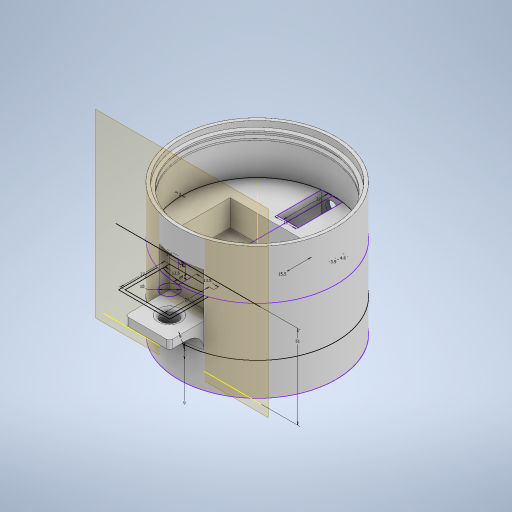
# Autodesk Inventor part: final_탄두_middle
Saved by Autodesk Inventor 2023 (Build 270158000, 158)
## iProperties
Created: 2023-10-31
Part Number: final_탄두_middle
Material: 일반
Document SubType Name: Modeling
Designer: rlatk
Density: 1 g/cm^3
Appearance: 기본값
Author: rlatk
Autodesk Inventor part; units mm, degrees
ref_plane "YZ Plane" through (0, 0, 0) normal (1, 0, 0) x (0, 1, 0)
ref_plane "XZ Plane" through (0, 0, 0) normal (0, 1, 0) x (-1, 0, 0)
sketch "스케치1" plane through (0, 0, 0) normal (0, 1, 0) x (-1, 0, 0)
  circle A0 centre (0, 0) radius 45.85
  circle A1 centre (0, 0) radius 47.85
  dimension "d0" = 91.7
  dimension "d1" = 2
  constraints: 2 centre point, 1 coincident
  measures "d0" diameter of A0
  measures "d1" radial gap between concentric circles of A0 A1
extrude "돌출1" add sketch "스케치1" along normal blind 10
ref_plane "작업 평면1" through (0, 0, 45.75) normal (0, 0, 1) x (1, 0, 0)
sketch "스케치2" plane through (0, 0, 45.75) normal (0, 0, 1) x (1, 0, 0)
  circle A0 centre (0, 9) radius 4.5
  line L0 (47.85, 0) -> (-47.85, 0) projected
  line L1 (-40.336, 51) -> (47.75, 51)
  line L2 (2, 52.9) -> (-2, 52.9)
  line L3 (-2, 52.9) -> (-2, 49.1)
  line L4 (-2, 49.1) -> (2, 49.1)
  line L5 (2, 49.1) -> (2, 52.9)
  line L6 (2, 52.9) -> (-2, 49.1) construction
  line L7 (-2, 52.9) -> (2, 49.1) construction
  point P0 (0, 0)
  point P1 (0, 51)
  dimension "d5" = 9
  dimension "d6" = 9
  dimension "d10" = 51
  dimension "d11" = 4
  dimension "d12" = 3.8
  constraints: 14 end point, 2 horizontal, 2 midpoint, 2 parallel, 1 centre point, 1 perpendicular, 1 point on line
  measures "d5" diameter of A0
  measures "d6" distance from line of L0 A0.centre
  measures "d10" distance between parallel lines of L1 L0
  measures "d11" distance of L4.end L3.end
  measures "d12" distance of L3.end L2.end
sketch "스케치3" plane through (0, 0, 0) normal (1, 0, 0) x (0, 1, 0)
  line L0 (10, 45.85) -> (0, 45.85) projected
  line L1 (-22.58, 0) -> (65.48, 0) projected
  line L2 (10, 45.85) -> (0, 45.85) projected
  line L3 (52.9, 45.85) -> (49.1, 45.85)
  line L4 (49.1, 45.85) -> (49.1, 44.85)
  line L5 (49.1, 44.85) -> (52.9, 44.85)
  line L6 (52.9, 44.85) -> (52.9, 45.85)
  point P0 (0, 0)
  point P1 (49.1, 45.75)
  point P2 (49.1, 45.75)
  point P3 (49.1, 45.75)
  point P4 (52.9, 45.75)
  point P5 (52.9, 45.75)
  point P6 (52.9, 45.75)
  dimension "d17" = 1
  constraints: 8 end point, 2 parallel, 1 horizontal, 1 perpendicular, 1 point on line, 1 other
  measures "d17" distance of L4.end L3.end
sketch "스케치4" plane through (0, 0, 0) normal (0, -1, 0) x (1, 0, 0)
  point P0 (0, 0)
sketch "스케치5" plane through (0, 0, 0) normal (0, -1, 0) x (1, 0, 0)
  circle A0 centre (0, 0) radius 45.85 projected
  circle A1 centre (0, 0) radius 47.85 projected
  circle A2 centre (0, 0) radius 45.85
  circle A3 centre (0, 0) radius 47.85
  constraints: 2 centre point, 2 coincident, 2 concentric
extrude "돌출4" add sketch "스케치5" along normal blind 10
sketch "스케치6" plane through (0, 0, 45.75) normal (0, 0, 1) x (1, 0, 0)
  point P0 (0, 0)
sketch "스케치7" plane through (0, 0, 0) normal (1, 0, 0) x (0, 1, 0)
  line L0 (10, 45.85) -> (-10, 45.85) projected
  line L1 (-9, 45.85) -> (-7, 45.85)
  line L2 (-7, 45.85) -> (-7, 43.85)
  line L3 (-7, 43.85) -> (-9, 43.85)
  line L4 (-9, 43.85) -> (-9, 45.85)
  line L5 (-9, 45.85) -> (-8.5, 43.85)
  line L6 (-7, 45.85) -> (-7.5, 43.85)
  point P0 (0, 0)
  dimension "d21" = 2
  dimension "d22" = 2
  dimension "d23" = 1
  dimension "d24" = 0.5
  dimension "d25" = 0.5
  constraints: 12 end point, 3 point on line, 2 parallel, 1 horizontal, 1 perpendicular
  measures "d21" distance of L2.end L3.end
  measures "d22" distance of L1.end L2.end
  measures "d23" distance of L1.start L0.end
  measures "d24" distance of L5.end L3.end
  measures "d25" distance of L2.end L6.end
coil "코일1" sketch "스케치7" operation add axis through (0, -10, 0) along (0, 1, 0) pitch 4 turns 2 hand right contours L6 L3 L5 L0
sketch "스케치8" plane through (0, 0, 0) normal (0, 0, 1) x (1, 0, 0)
  line L0 (-47.85, -10) -> (47.85, -10) projected
  line L1 (47.85, 10) -> (-47.85, 10) projected
  point P0 (0, 0)
sketch "스케치9" plane through (0, 10, 0) normal (0, 1, 0) x (1, 0, 0)
  circle A0 centre (0, 0) radius 47.85 projected
  circle A1 centre (0, 0) radius 45.85 projected
  circle A2 centre (0, 0) radius 47.85
  constraints: 1 centre point, 1 coincident, 1 concentric
extrude "돌출5" add sketch "스케치9" along normal blind 30 contours A0 | A1
sketch "스케치10" plane through (0, 40, 0) normal (0, 1, 0) x (1, 0, 0)
  circle A0 centre (0, 0) radius 47.85 projected
  circle A1 centre (0, 0) radius 45.85
  circle A2 centre (0, 0) radius 47.85
  line L0 (0, -47.85) -> (0, 47.85)
  line L1 (-6.5, 45.3869) -> (-6.5, 18.3869)
  line L2 (-6.5, 18.3869) -> (6.5, 18.3869)
  circle A3 centre (0, 0) radius 45.85 projected
  line L3 (0, 45.85) -> (-0.1096, 45.3869) construction
  line L4 (0, 45.85) -> (0.1096, 45.3869) construction
  line L5 (-6.5, 45.3869) -> (6.5, 45.3869)
  line L6 (6.5, 18.3869) -> (6.5, 45.3869)
  dimension "d36" = 2
  dimension "d37" = 13
  dimension "d39" = 27
  constraints: 14 end point, 5 point on circle, 3 point on line, 2 centre point, 1 coincident, 1 parallel, 1 vertical
  measures "d36" radial gap between concentric circles of A0 A1
  measures "d37" distance of L2.end L1.end
  measures "d39" distance between parallel lines of L5 L2
extrude "돌출6" cut sketch "스케치10" against normal blind 27 contours L6 L2 L0 L5 | L5 L0 L2 L1
sketch "스케치11" plane through (0, 13, 0) normal (0, 1, 0) x (1, 0, 0)
  line L0 (-6.5, 45.3869) -> (6.5, 45.3869) projected
  line L1 (-6.5, 18.3869) -> (-6.5, 45.3869) projected
  line L2 (6.5, 18.3869) -> (-6.5, 18.3869) projected
  line L3 (6.5, 45.3869) -> (6.5, 18.3869) projected
  line L4 (-6.5, 18.3869) -> (-6.5, 45.3869) projected
  line L5 (-6.5, 45.3869) -> (6.5, 45.3869)
  line L6 (6.5, 45.3869) -> (6.5, 40.7869)
  line L7 (6.5, 40.7869) -> (-6.5, 40.7869)
  line L8 (-6.5, 40.7869) -> (-6.5, 45.3869)
  line L9 (-6.5, 33.8869) -> (6.5, 33.8869)
  line L10 (-6.5, 36.8869) -> (6.5, 36.8869)
  point P0 (0, 0)
  dimension "d42" = 4.6
  dimension "d43" = 15.5
  dimension "d44" = 3.9
  constraints: 12 end point, 5 point on line, 3 perpendicular, 2 parallel, 1 horizontal
  measures "d42" distance of L5.end L6.end
  measures "d43" distance between parallel lines of L2 L9
  measures "d44" distance between parallel lines of L10 L7
extrude "돌출10" add sketch "스케치9" against normal blind 5 contours A1
extrude "돌출12" cut sketch "스케치11" against normal blind 5.2 contours L10 L3 L9 L1
extrude "돌출13" add sketch "스케치11" along normal blind 7.8 contours L0 L3 L7 L1
sketch "스케치12" plane through (-6.5, 40, -45.3869) normal (0, 0, 1) x (1, 0, 0)
  point P0 (6.5, -40)
sketch "스케치13" plane through (-6.5, 40, -45.3869) normal (0, 0, 1) x (1, 0, 0)
  line L0 (54.35, 0) -> (-41.35, 0) projected
  line L1 (-41.35, -50) -> (54.35, -50) projected
  line L2 (0, -19.2) -> (13, -19.2) projected
  line L3 (13, 0) -> (13, -19.2) projected
  line L4 (0, 0) -> (13, 0) projected
  line L5 (0, 0) -> (0, -19.2) projected
  line L6 (0, -19.2) -> (13, -19.2) projected
  line L7 (0, -19.2) -> (13, -19.2) projected
  line L8 (13, -27) -> (0, -27) projected
  line L9 (13, -19.2) -> (13, -27) projected
  line L10 (0, -19.2) -> (13, -19.2) projected
  line L11 (0, -27) -> (0, -19.2) projected
  circle A0 centre (6.5, -6.3) radius 3.7
  point P0 (6.5, -40)
  dimension "d59" = 7.4
  dimension "d60" = 6.3
  constraints: 1 centre point
  measures "d59" diameter of A0
  measures "d60" distance from line of A0.centre L0
extrude "돌출14" cut sketch "스케치13" against normal blind 7.8 contours A0
sketch "스케치14" plane through (0, 40, 0) normal (0, 1, 0) x (1, 0, 0)
  line L0 (-6.5, 18.3869) -> (-6.5, 45.3869) projected
  line L1 (-6.5, 45.3869) -> (6.5, 45.3869) projected
  line L2 (6.5, 45.3869) -> (6.5, 18.3869) projected
  line L3 (6.5, 18.3869) -> (-6.5, 18.3869) projected
  circle A0 centre (0, 0) radius 47.85 projected
  line L4 (0, 0) -> (0, -47.85)
  line L5 (30, 13.5566) -> (-30, 13.5566)
  line L6 (-30, 13.5566) -> (-30, -26.4434)
  line L7 (-30, -26.4434) -> (30, -26.4434)
  line L8 (30, -26.4434) -> (30, 13.5566)
  line L9 (30, 13.5566) -> (-30, -26.4434) construction
  line L10 (-30, 13.5566) -> (30, -26.4434) construction
  point P0 (0, -6.4434)
  dimension "d63" = 60
  dimension "d64" = 40
  constraints: 14 end point, 2 midpoint, 2 parallel, 1 horizontal, 1 perpendicular, 1 point on line, 1 vertical alignment, 1 other
  measures "d63" distance of L7.end L6.end
  measures "d64" distance of L6.end L5.end
extrude "돌출15" cut sketch "스케치14" against normal blind 16 contours L8 L7 L6 L5
extrude "돌출16" add sketch "스케치10" along normal blind 30 contours A0 L0 A1 | L0 A1 A0
sketch "스케치15" plane through (0, 0, 45.75) normal (0, 0, 1) x (1, 0, 0)
  point P0 (0, 0)
sketch "스케치16" plane through (0, 0, 0) normal (1, 0, 0) x (0, 1, 0)
  line L0 (5, -45.85) -> (5, 45.85) projected
  line L1 (-1, 45.85) -> (1, 45.85) projected
  line L2 (-7, 45.85) -> (-9, 45.85) projected
  line L3 (-10, -45.85) -> (-10, 45.85) projected
  line L4 (70, 45.85) -> (40, 45.85) projected
  line L5 (58, 45.85) -> (58, 43.85)
  line L6 (58, 43.85) -> (60, 43.85)
  line L7 (60, 43.85) -> (60, 45.85)
  line L8 (59, 45.85) -> (58, 43.85) construction
  line L9 (59, 45.85) -> (60, 43.85) construction
  line L10 (60, 45.85) -> (58, 45.85)
  line L11 (60, 45.85) -> (59.5, 43.85)
  line L12 (58, 45.85) -> (58.5, 43.85)
  point P0 (0, 0)
  dimension "d69" = 11
  dimension "d70" = 2
  dimension "d72" = 0.5
  dimension "d73" = 0.5
  constraints: 16 end point, 3 point on line, 2 horizontal alignment, 1 midpoint, 1 parallel
  measures "d69" distance of L8.start L4.start
  measures "d70" distance of L6.end L5.end
  measures "d72" distance of L5.end L12.end
  measures "d73" distance of L11.end L6.end
coil "코일2" sketch "스케치16" operation add axis through (0, -10, 0) along (0, 1, 0) pitch 4 turns 2 hand right contours L11 L6 L12 L4
sketch "스케치17" plane through (0, 70, 0) normal (0, 1, 0) x (1, 0, 0)
  point P0 (0, 0)
sketch "스케치18" plane through (0, -10, 0) normal (0, -1, 0) x (1, 0, 0)
  circle A0 centre (0, 0) radius 47.85 projected
  circle A1 centre (0, 0) radius 45.85 projected
  circle A2 centre (0, 0) radius 47.85
  circle A3 centre (0, 0) radius 45.85
  constraints: 2 centre point, 2 coincident, 1 concentric
sketch "스케치19" plane through (0, 40, 0) normal (0, 1, 0) x (1, 0, 0)
  circle A0 centre (0, 0) radius 45.85 projected
  circle A1 centre (0, 0) radius 47.85 projected
  line L0 (0, -47.85) -> (0, 47.85) projected
  line L1 (0, -47.85) -> (0, -39.85)
  line L2 (0, -39.85) -> (-13.5, -39.85)
  line L3 (0, -39.85) -> (13.5, -39.85)
  line L4 (-13.5, -39.85) -> (-13.5, -66.85)
  line L5 (13.5, -39.85) -> (13.5, -66.85)
  line L6 (13.5, -66.85) -> (-13.5, -66.85)
  line L7 (-15.5, -68.85) -> (-15.5, -37.85)
  line L8 (-15.5, -37.85) -> (0, -37.85)
  line L9 (0, -37.85) -> (15.5, -37.85)
  line L10 (15.5, -37.85) -> (15.5, -68.85)
  line L11 (15.5, -68.85) -> (-15.5, -68.85)
  circle A2 centre (0, -53.35) radius 5
  point P0 (13.5, -45.9061)
  point P1 (-13.5, -45.9061)
  point P2 (-13.5, -43.8175)
  point P3 (13.5, -43.8175)
  point P4 (-15.5, -43.1506)
  point P5 (15.5, -43.1506)
  dimension "d82" = 8
  dimension "d83" = 13.5
  dimension "d84" = 13.5
  dimension "d85" = 27
  dimension "d86" = 27
  dimension "d87" = 2
  dimension "d88" = 10
  constraints: 22 end point, 2 vertical, 1 centre point, 1 horizontal, 1 perpendicular, 1 point on line, 4 other
  measures "d82" distance of L0.start L1.end
  measures "d83" distance of L1.end L2.end
  measures "d84" distance of L1.end L3.end
  measures "d85" distance of L2.end L4.end
  measures "d86" distance of L3.end L5.end
  measures "d87" distance between parallel lines of L4 L7
  measures "d88" diameter of A2
extrude "돌출18" cut sketch "스케치19" along normal blind 13.5 and the other way blind 13.5 contours L5 A1 L0 A0 | A0 L0 L3 L5 | L4 L2 L0 A0 | A0 L0 A1 L4
extrude "돌출19" add sketch "스케치19" along normal blind 13.5 contours A0 L5 L3 L0 L9 L10 | L7 L8 L0 L2 L4 A0
sketch "스케치20" plane through (0, 53.5, 0) normal (0, 1, 0) x (1, 0, 0)
  line L0 (-15.5, -68.85) -> (-15.5, -37.85) projected
  line L1 (-13.5, -39.85) -> (-13.5, -66.85) projected
  line L2 (-15.5, -37.85) -> (0, -37.85) projected
  line L3 (-15.5, -37.85) -> (15.5, -37.85) projected
  line L4 (0, -39.85) -> (13.5, -39.85) projected
  line L5 (0, -39.85) -> (-13.5, -39.85) projected
  line L6 (13.5, -39.85) -> (13.5, -66.85) projected
  line L7 (15.5, -37.85) -> (15.5, -43.1506) projected
  line L8 (15.5, -37.85) -> (15.5, -68.85) projected
  circle A0 centre (0, 0) radius 47.85 projected
  point P0 (15.5, -45.27)
  point P1 (-15.5, -45.27)
extrude "돌출20" add sketch "스케치20" along normal blind 2 contours L0 L2 L3 L7 L8 A0 L6 L4 L5 L1 | L1 L5 L4 L6 A0
sketch "스케치21" plane through (0, 26.5, 0) normal (0, 1, 0) x (1, 0, 0)
  line L0 (-15.5, -68.85) -> (-15.5, -37.85) projected
  line L1 (15.5, -68.85) -> (-15.5, -68.85) projected
  line L2 (15.5, -37.85) -> (15.5, -68.85) projected
  line L3 (13.5, -39.85) -> (13.5, -66.85) projected
  line L4 (15.5, -37.85) -> (-15.5, -37.85) projected
  line L5 (-13.5, -39.85) -> (13.5, -39.85) projected
  line L6 (-13.5, -39.85) -> (-13.5, -66.85) projected
  line L7 (13.5, -66.85) -> (-13.5, -66.85) projected
  circle A0 centre (0, -53.35) radius 5 projected
  point P0 (0, 0)
extrude "돌출21" add sketch "스케치21" against normal blind 5 contours L3 L7 L6 L5
fillet "모깎기2" radius 10 1 edges at (0, 21.5, 47.85)
fillet "모깎기3" radius 2 6 edges at (-13.5, 24, 66.85) (13.5, 24, 66.85) (-5, 26.5, 53.35) (0, 21.5, 58.35) (-2.1069, 15.8816, 48.8156) (4.3208, 21.3335, 55.8661)
